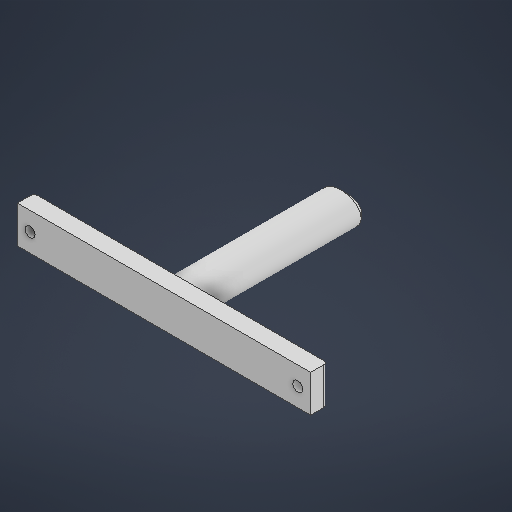
# Autodesk Inventor part: apoioG
Saved by Autodesk Inventor 2026 (Build 300175050, 175E)
## iProperties
Created: 2025-06-11
Part Number: apoioG
Material: Generic
Document SubType Name: Modeling
Designer: dcana
Density: 1 g/cm^3
Appearance: Default
Author: dcana
Autodesk Inventor part; units mm, degrees
ref_plane "YZ Plane" through (0, 0, 0) normal (1, 0, 0) x (0, 1, 0)
ref_plane "XZ Plane" through (0, 0, 0) normal (0, 1, 0) x (-1, 0, 0)
ref_plane "XY Plane" through (0, 0, 0) normal (0, 0, 1) x (1, 0, 0)
sketch "Sketch1" plane through (0, 0, 0) normal (0, 0, 1) x (1, 0, 0)
  line L0 (-40, 0) -> (40, 0)
  circle A0 centre (-40, 0) radius 1.5
  circle A1 centre (40, 0) radius 1.5
  line L1 (-43.8161, 5.5412) -> (43.8161, 5.5412)
  line L2 (43.8161, 5.5412) -> (43.8161, -5.5412)
  line L3 (43.8161, -5.5412) -> (-43.8161, -5.5412)
  line L4 (-43.8161, -5.5412) -> (-43.8161, 5.5412)
  ellipse E0 centre (-0.0839, -0.042) end of major axis (-6.111, -0.042) minor radius 4.3359
  point P0 (0, 0)
  point P1 (0, 0)
  point P2 (0, -5.5412)
  point P3 (-43.8161, 0)
  point P4 (43.8161, 0)
  constraints: 10 end point, 4 midpoint, 2 centre point, 2 coincident, 2 horizontal, 2 parallel, 1 perpendicular, 2 other
extrude "Extrusion2" add sketch "Sketch1" along normal blind 5
sketch "Sketch4" plane through (0, 0, 0) normal (0, 0, -1) x (-1, 0, 0)
  ellipse E0 centre (0.0839, -0.042) end of major axis (-5.9431, -0.042) minor radius 4.3359 projected
  point P0 (0, 0)
  constraints: 1 other
extrude "Extrusion3" add sketch "Sketch4" along normal blind 50 and the other way blind 5
chamfer "Chamfer1" distance 2 angle 45 1 edges at (-6.111, -0.042, -50)
fillet "Fillet1" radius 1 1 edges at (-43.8161, 0, 0)
fillet "Fillet2" radius 1 1 edges at (43.8161, 0, 0)
body "Solid2"
